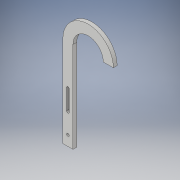
# Autodesk Inventor part: ScissorHookTry
Saved by Autodesk Inventor 2018 (Build 220112000, 112)
## iProperties
Created: 2020-01-27
Part Number: ScissorHookTry
Material: Generic
Document SubType Name: Modeling
Designer: Myers
Mass: 60.1611 g
Surface Area: 250.995 cm^2
Volume: 60.1611 cm^3
Density: 1 g/cm^3
Appearance: Default
Author: Myers
Autodesk Inventor part; units mm, degrees
ref_plane "YZ Plane" through (0, 0, 0) normal (1, 0, 0) x (0, 1, 0)
ref_plane "XZ Plane" through (0, 0, 0) normal (0, 1, 0) x (-1, 0, 0)
ref_plane "XY Plane" through (0, 0, 0) normal (0, 0, 1) x (1, 0, 0)
sketch "Sketch1" plane through (0, 0, 0) normal (0, 0, 1) x (1, 0, 0)
  line L0 (12.7, 127) -> (12.7, -101.6)
  line L1 (12.7, -101.6) -> (-12.7, -101.6)
  line L2 (-12.7, -101.6) -> (-12.7, 127)
  arc A0 (88.9, 127) -> (12.7, 127) centre (50.8, 127) ccw
  arc A1 (114.3, 127) -> (-12.7, 127) centre (50.8, 127) ccw
  line L3 (88.9, 127) -> (114.3, 127)
  point P0 (0, 588.8574)
  point P1 (0, -101.6)
  dimension "d6" = 25.4
  dimension "d7" = 38.1
  constraints: 8 end point, 4 point on circle, 2 centre point, 2 tangent, 1 concentric, 1 horizontal, 1 midpoint, 1 parallel, 1 point on line
  measures "d6" distance of L0.end L1.end
  measures "d7" radius of A0
extrude "Extrusion1" add sketch "Sketch1" along normal blind 9.525
sketch "Sketch3" plane through (0, 0, 9.525) normal (0, 0, 1) x (1, 0, 0)
  line L0 (-12.7, 127) -> (-12.7, -101.6) projected
  line L1 (-12.7, -101.6) -> (12.7, -101.6) projected
  line L2 (12.7, -101.6) -> (12.7, 127) projected
  arc A0 (88.9, 127) -> (12.7, 127) centre (50.8, 127) ccw projected
  line L3 (88.9, 127) -> (114.3, 127) projected
  arc A1 (114.3, 127) -> (-12.7, 127) centre (50.8, 127) ccw projected
  point P0 (0, 0)
  point P1 (0, -76.2)
  dimension "d20" = 12.7
  dimension "d21" = 12.7
  dimension "d22" = 25.4
  measures "d20" distance from line of L0 point (0, -76.2)
  measures "d21" distance from line of L2 point (0, -76.2)
  measures "d22" distance from line of L1 point (0, -76.2)
hole "Hole1" at (0, -76.2, 9.525) direction (0, 0, -1) diameter 6.7564 end through all clearance for "Flat Head Machine Screw (82)" size "1/4" standard "Ansi Unified Screw Threads"
sketch "Sketch4" plane through (0, 0, 9.525) normal (0, 0, 1) x (1, 0, 0)
  circle A0 centre (0, -76.2) radius 3.3782 projected
  line L0 (-12.7, 127) -> (-12.7, -101.6) projected
  line L1 (-12.7, -101.6) -> (12.7, -101.6) projected
  line L2 (12.7, -101.6) -> (12.7, 127) projected
  arc A1 (88.9, 127) -> (12.7, 127) centre (50.8, 127) ccw projected
  line L3 (88.9, 127) -> (114.3, 127) projected
  arc A2 (114.3, 127) -> (-12.7, 127) centre (50.8, 127) ccw projected
  line L4 (-3.3782, -25.4) -> (-3.3782, 25.4)
  line L5 (3.3782, 25.4) -> (3.3782, -25.4)
  circle A3 centre (0, -76.2) radius 3.3782 projected
  arc A4 (3.3782, 25.4) -> (-3.3782, 25.4) centre (0, 25.4) ccw
  arc A5 (-3.3782, -25.4) -> (3.3782, -25.4) centre (0, -25.4) ccw
  point P0 (0, 0)
  dimension "d23" = 50.8
  dimension "d24" = 50.8
  constraints: 6 tangent, 4 end point, 4 point on circle, 2 centre point, 2 vertical
  measures "d23" distance of A5.centre A4.centre
  measures "d24" distance of A0.centre A5.centre
extrude "Extrusion2" cut sketch "Sketch4" against normal through all contours L4 A4 L5 A5
equation "\"d20\" = d21"
body "Solid1"
